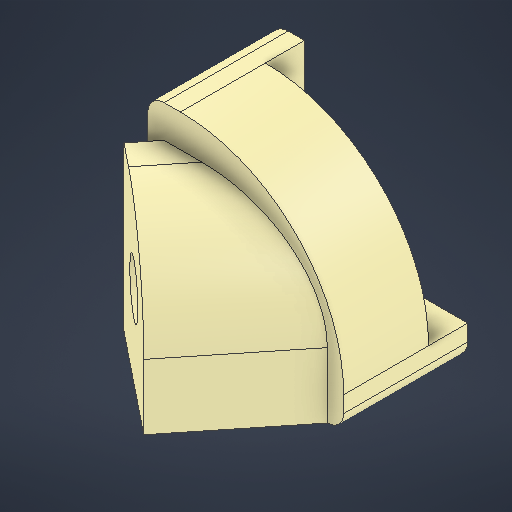
# Autodesk Inventor part: display_bottom_support_right
Saved by Autodesk Inventor 2026 (Build 300175050, 175E)
## iProperties
Created: 2025-06-09
Part Number: display_bottom_support_right
Material: Generic
Document SubType Name: Modeling
Designer: satom
Density: 1 g/cm^3
Appearance: Default
Author: satom
Autodesk Inventor part; units mm, degrees
ref_plane "YZ Plane" through (0, 0, 0) normal (1, 0, 0) x (0, 1, 0)
ref_plane "XZ Plane" through (0, 0, 0) normal (0, 1, 0) x (-1, 0, 0)
ref_plane "XY Plane" through (0, 0, 0) normal (0, 0, 1) x (1, 0, 0)
sketch "Sketch2" plane through (0, 0, 0) normal (0, 0, 1) x (1, 0, 0)
  line L0 (0, 0) -> (12.7, 0)
  line L1 (0, 0) -> (0, 12.7)
  arc A0 (12.7, 0) -> (0, 12.7) centre (0, 0) ccw
  circle A1 centre (5.08, 5.08) radius 3.1115
  dimension "d4" = 12.7
  dimension "d5" = 6.223
  dimension "d6" = 5.08
  dimension "d7" = 5.08
  constraints: 4 end point, 2 centre point, 2 coincident, 2 point on circle, 1 horizontal, 1 vertical
  measures "d4" distance of L0.start L1.end
  measures "d5" diameter of A1
  measures "d6" distance from line of L0 A1.centre
  measures "d7" distance from line of L1 A1.centre
extrude "Extrusion1" add sketch "Sketch2" along normal blind 3.81
sketch "Sketch4" plane through (0, 0, 0) normal (0, 0, -1) x (-1, 0, 0)
  arc A0 (0, 12.7) -> (-12.7, 0) centre (0, 0) ccw projected
  line L0 (-12.7, 0) -> (-12.7, -1.27)
  line L1 (0, 12.7) -> (1.27, 12.7)
  line L2 (2.54, 11.43) -> (2.54, -1.27)
  line L3 (1.27, -2.54) -> (-11.43, -2.54)
  line L4 (0, 12.7) -> (0, 0)
  line L5 (0, 0) -> (-12.7, 0)
  arc A1 (-12.7, -1.27) -> (-11.43, -2.54) centre (-11.43, -1.27) ccw
  arc A2 (1.27, -2.54) -> (2.54, -1.27) centre (1.27, -1.27) ccw
  arc A3 (2.54, 11.43) -> (1.27, 12.7) centre (1.27, 11.43) ccw
  point P0 (-12.7, -2.54)
  point P1 (2.54, 12.7)
  dimension "d10" = 2.54
  dimension "d11" = 2.54
  dimension "d12" = 1.27
  constraints: 12 end point, 7 tangent, 6 point on circle, 4 perpendicular, 4 point on line, 3 centre point, 2 equal radius, 1 horizontal, 1 vertical
  measures "d10" distance of L0.start point (-12.7, -2.54)
  measures "d11" distance of L1.start point (2.54, 12.7)
  measures "d12" radius of A1
extrude "Extrusion2" add sketch "Sketch4" along normal blind 3.048 and the other way blind 3.81 contours L1 A3 L2 A2 L3 A1 L0 L5 L4
sketch "Sketch5" plane through (0, 0, 3.81) normal (0, 0, 1) x (1, 0, 0)
  line L0 (-1.27, -2.54) -> (11.43, -2.54)
  line L1 (-2.54, -1.27) -> (-2.54, 11.43)
  arc A0 (12.7, 0) -> (0, 12.7) centre (0, 0) ccw
  line L2 (0, 12.7) -> (-1.27, 12.7)
  line L3 (12.7, 0) -> (12.7, -1.27)
  arc A1 (-1.27, 12.7) -> (-2.54, 11.43) centre (-1.27, 11.43) ccw
  arc A2 (-2.54, -1.27) -> (-1.27, -2.54) centre (-1.27, -1.27) ccw
  arc A3 (11.43, -2.54) -> (12.7, -1.27) centre (11.43, -1.27) ccw
  line L4 (0, 12.7) -> (0, 0) projected
  line L5 (0, 0) -> (12.7, 0) projected
  circle A4 centre (5.08, 5.08) radius 3.1115
  dimension "d17" = 1.27
  dimension "d18" = 2.54
  dimension "d19" = 2.54
  constraints: 8 end point, 8 point on circle, 6 tangent, 5 centre point, 2 equal radius, 2 horizontal, 1 coincident, 1 perpendicular, 1 vertical
  measures "d17" radius of A1
  measures "d18" distance between parallel lines of L1 L4
  measures "d19" distance between parallel lines of L5 L0
extrude "Extrusion3" add sketch "Sketch5" along normal blind 2.794 contours A2 L1 A1 L2 L4 L5 L3 A3 L0 | L5 L4 A0 | A4
sketch "Sketch7" plane through (-1.27, -2.54, -3.048) normal (0, -1, 0) x (1, 0, 0)
  line L0 (12.7, 0) -> (12.7, 9.652) projected
  line L1 (12.7, 9.652) -> (6.3503, 17.5834)
  line L2 (0, 9.652) -> (0, 0) projected
  line L3 (0, 9.652) -> (-1.3892, 11.3873)
  line L4 (6.3503, 17.5834) -> (-1.3892, 11.3873)
  line L5 (12.7, 9.652) -> (0, 9.652)
  point P0 (1.27, 3.048)
  dimension "d22" = 141.32
  dimension "d23" = 141.32
  dimension "d24" = 10.16
  constraints: 8 end point, 1 horizontal, 1 perpendicular
  measures "d22" angle of L0 L1
  measures "d23" angle of L2 L3
  measures "d24" distance of L0.end L1.end
extrude "Extrusion4" add sketch "Sketch7" against normal blind 12.7
sketch "Sketch8" plane through (5.0803, -2.54, 14.5354) normal (-0.6249702, 0, 0.7806486) x (0.7806486, 0, 0.6249702)
  line L0 (0, 0) -> (-9.9142, 0) construction
  line L1 (-9.9142, 12.7) -> (0, 12.7) construction
  line L2 (0, 0) -> (-9.9142, 12.7) construction
  line L3 (-9.9142, 0) -> (-9.9142, 12.7) construction
  line L4 (-9.9142, 0) -> (-1.8469, 10.3341) construction
  circle A0 centre (-4.9571, 6.35) radius 2
  point P0 (-13.0501, 2.54)
  dimension "d27" = 4
  constraints: 4 end point, 1 centre point, 1 midpoint, 1 point on line
  measures "d27" diameter of A0
extrude "Extrusion5" cut sketch "Sketch8" against normal blind 7
fillet "Fillet1" radius 7.62 1 edges at (8.2552, 10.16, 10.5697)
equation "\"d27\" = m3_heat_set_insert"
equation "\"d28\" = m3_heat_set_depth"
equation "\"m3_heat_set_insert\" = 4"
equation "\"m3_clearance\" = 3.4"
equation "\"m3_heat_set_depth\" = 7"
equation "\"robot_diameter\" = 354"
equation "\"hardboard_thickness\" = 5"
body "Solid1"
